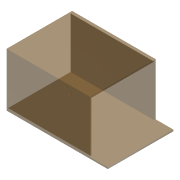
# Autodesk Inventor part: Bucket
Saved by Autodesk Inventor 2015 (Build 190159000, 159)
## iProperties
Created: 2015-01-24
Part Number: Bucket
Material: Generic
Document SubType Name: Modeling
Designer: rihoobler
Density: 1 g/cm^3
Appearance: Polycarbonate - Smoked
Author: rihoobler
Autodesk Inventor part; units mm, degrees
ref_plane "YZ Plane" through (0, 0, 0) normal (1, 0, 0) x (0, 1, 0)
ref_plane "XZ Plane" through (0, 0, 0) normal (0, 1, 0) x (-1, 0, 0)
ref_plane "XY Plane" through (0, 0, 0) normal (0, 0, 1) x (1, 0, 0)
sketch "Sketch1" plane through (0, 0, 0) normal (1, 0, 0) x (0, 1, 0)
  line L0 (0, 0) -> (114.3, 0)
  line L1 (114.3, 0) -> (114.3, -139.7)
  line L2 (114.3, -139.7) -> (0, -139.7)
  line L3 (0, -139.7) -> (0, 0)
  line L4 (111.125, -136.525) -> (111.125, -3.175)
  line L5 (111.125, -3.175) -> (3.175, -3.175)
  line L6 (3.175, -3.175) -> (3.175, -136.525)
  line L7 (3.175, -136.525) -> (111.125, -136.525)
  dimension "d0" = 114.3
  dimension "d1" = 139.7
  dimension "d2" = 3.175
  constraints: 16 end point, 4 parallel, 2 perpendicular, 1 horizontal, 3 other
  measures "d0" distance of L1.end L2.end
  measures "d1" distance of L0.end L1.end
  measures "d2" distance between parallel lines of L0 L5
extrude "Extrusion1" add sketch "Sketch1" along normal blind 215.9
sketch "Sketch2" plane through (0, 0, 0) normal (0, 0, 1) x (1, 0, 0)
  line L0 (215.9, 114.3) -> (177.8, 114.3)
  line L1 (177.8, 114.3) -> (177.8, 3.175)
  line L2 (177.8, 3.175) -> (215.9, 3.175)
  line L3 (215.9, 3.175) -> (215.9, 114.3)
  point P0 (0, 0)
  dimension "d5" = 38.1
  dimension "d6" = 111.125
  constraints: 8 end point, 2 parallel, 1 horizontal, 1 perpendicular
  measures "d5" distance of L2.end L1.end
  measures "d6" distance of L1.end L0.end
extrude "Extrusion2" cut sketch "Sketch2" against normal through all
sketch "Sketch4" plane through (0, 0, 0) normal (0, 0, 1) x (1, 0, 0)
  line L0 (177.8, 3.175) -> (177.8, 114.3) projected
  line L1 (0, 114.3) -> (177.8, 114.3) projected
  circle A0 centre (127, 97.79) radius 4
  line L2 (127, 97.79) -> (134.9404, 98.765)
  line L3 (127, 97.79) -> (135, 97.79) construction
  line L4 (127, 97.79) -> (126.025, 105.7304)
  circle A1 centre (126.025, 105.7304) radius 1.85
  circle A2 centre (134.9404, 98.765) radius 1.85
  dimension "d13" = 50.8
  dimension "d14" = 16.51
  dimension "d15" = 8
  dimension "d16" = 8
  dimension "d17" = 353
  dimension "d18" = 8
  dimension "d19" = 3.7
  dimension "d20" = 3.7
  dimension "d23" = 90
  constraints: 6 end point, 3 centre point, 3 coincident, 1 equal length, 1 horizontal
  measures "d13" distance from line of L0 point (127, 97.79)
  measures "d14" distance from line of L1 point (127, 97.79)
  measures "d15" diameter of A0
  measures "d16" distance of L2.start L2.end
  measures "d18" distance of L2.start L4.end
  measures "d19" diameter of A1
  measures "d20" diameter of A2
  measures "d23" angle of L2 L4
extrude "Extrusion3" cut sketch "Sketch4" against normal blind 25.4 contours A1 | A2
body "Solid1"
